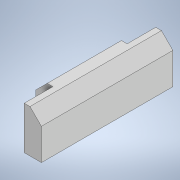
# Autodesk Inventor part: outside-join
Saved by Autodesk Inventor 2021 (Build 250183000, 183)
## iProperties
Created: 2020-12-08
Part Number: outside-join
Material: Generic
Document SubType Name: Modeling
Designer: Luke Kamols
Density: 1 g/cm^3
Appearance: Default
Author: Luke Kamols
Autodesk Inventor part; units mm, degrees
ref_plane "YZ Plane" through (0, 0, 0) normal (1, 0, 0) x (0, 1, 0)
ref_plane "XZ Plane" through (0, 0, 0) normal (0, 1, 0) x (-1, 0, 0)
ref_plane "XY Plane" through (0, 0, 0) normal (0, 0, 1) x (1, 0, 0)
sketch "Sketch1" plane through (0, 0, 0) normal (0, 0, 1) x (1, 0, 0)
  line L0 (0, 0) -> (6, 0)
  line L1 (6, 0) -> (6, 11)
  line L2 (0, 0) -> (0, 15)
  line L3 (0, 15) -> (2, 15)
  line L4 (2, 15) -> (6, 11)
  dimension "d0" = 6
  dimension "d1" = 11
  dimension "d2" = 15
  dimension "d3" = 2
  constraints: 10 end point, 2 perpendicular, 1 horizontal, 1 vertical
  measures "d0" distance of L0.start L0.end
  measures "d1" distance of L0.end L1.end
  measures "d2" distance of L0.start L2.end
  measures "d3" distance of L2.end L3.end
extrude "Extrusion1" add sketch "Sketch1" along normal blind 10
sketch "Sketch2" plane through (0, 0, 10) normal (0, 0, 1) x (1, 0, 0)
  line L0 (0, 15) -> (0, 0) projected
  line L1 (0, 0) -> (6, 0) projected
  line L2 (6, 11) -> (2, 15) projected
  line L3 (0, 11) -> (3, 8)
  line L4 (0, 11) -> (-3, 8)
  line L5 (-3, 8) -> (-3, 0)
  line L6 (2, 15) -> (0, 15) projected
  line L7 (0, 15) -> (2, 15)
  line L8 (6, 0) -> (6, 11) projected
  line L9 (2, 15) -> (6, 11)
  line L10 (6, 11) -> (6, 0)
  line L11 (6, 0) -> (0, 0)
  line L12 (0, 0) -> (-6, 0)
  line L13 (-6, 11) -> (-2, 15)
  line L14 (-2, 15) -> (0, 15)
  line L15 (-6, 0) -> (-6, 11)
  line L16 (3, 8) -> (3, 0)
  line L17 (3, 0) -> (6, 0)
  line L18 (-3, 0) -> (-6, 0)
  line L19 (0, 11) -> (0, 15)
  dimension "d6" = 3
  constraints: 30 end point, 5 collinear, 3 symmetric about line, 2 vertical, 1 horizontal, 1 midpoint, 1 perpendicular, 1 point on line
  measures "d6" distance of L0.end L16.end
extrude "Extrusion2" add sketch "Sketch2" along normal blind 26 contours L6 L2 L8 L1 L16 L3 L0 | L0 L4 L5 L12 L15 L13 L14
sketch "Sketch3" plane through (0, 0, 36) normal (0, 0, 1) x (1, 0, 0)
  line L0 (2, 15) -> (-2, 15) projected
  line L1 (0, 15) -> (2, 15)
  line L2 (6, 11) -> (2, 15) projected
  line L3 (2, 15) -> (6, 11)
  line L4 (6, 0) -> (6, 11) projected
  line L5 (6, 11) -> (6, 0)
  line L6 (0, 0) -> (6, 0) projected
  line L7 (6, 0) -> (0, 0)
  line L8 (0, 15) -> (0, 11) projected
  line L9 (0, 0) -> (0, 15)
  constraints: 10 end point, 4 collinear, 1 perpendicular
extrude "Extrusion3" add sketch "Sketch3" along normal blind 10
body "Solid1"
